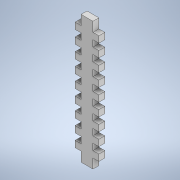
# Autodesk Inventor part: cover
Saved by Autodesk Inventor 2020 (Build 240168000, 168)
## iProperties
Created: 2019-12-19
Part Number: cover
Material: Générique
Document SubType Name: Modeling
Designer: damien
Density: 1 g/cm^3
Appearance: Par défaut
Author: damien
Autodesk Inventor part; units mm, degrees
ref_plane "YZ Plane" through (0, 0, 0) normal (1, 0, 0) x (0, 1, 0)
ref_plane "XZ Plane" through (0, 0, 0) normal (0, 1, 0) x (-1, 0, 0)
ref_plane "XY Plane" through (0, 0, 0) normal (0, 0, 1) x (1, 0, 0)
sketch "Esquisse1" plane through (0, 0, 0) normal (0, 0, 1) x (1, 0, 0)
  line L0 (37.1, -200) -> (-37.1, -200)
  line L1 (-37.1, -200) -> (-37.1, 200)
  line L2 (-37.1, 200) -> (37.1, 200)
  line L3 (37.1, 200) -> (37.1, -200)
  line L4 (37.1, -200) -> (-37.1, 200) construction
  line L5 (-37.1, -200) -> (37.1, 200) construction
  point P0 (0, 0)
  dimension "d0" = 400
  dimension "d1" = 74.2
  constraints: 12 end point, 2 midpoint, 2 parallel, 1 horizontal, 1 perpendicular
  measures "d0" distance of L0.end L1.end
  measures "d1" distance of L0.start L0.end
extrude "Extrusion1" add sketch "Esquisse1" along normal blind 18.55
sketch "Esquisse2" plane through (0, 0, 18.55) normal (0, 0, 1) x (1, 0, 0)
  line L0 (-37.1, 200) -> (-37.1, -200) projected
  line L1 (-37.1, 150) -> (-18.55, 150)
  line L2 (-18.55, 150) -> (-18.55, 130)
  line L3 (-18.55, 130) -> (-37.1, 130)
  line L4 (-37.1, 130) -> (-37.1, 150)
  line L5 (37.1, 200) -> (-37.1, 200) projected
  line L6 (-37.1, 90) -> (-37.1, 110)
  line L7 (-37.1, 110) -> (-18.55, 110)
  line L8 (-18.55, 110) -> (-18.55, 90)
  line L9 (-18.55, 90) -> (-37.1, 90)
  line L10 (-37.1, 50) -> (-37.1, 70)
  line L11 (-37.1, 70) -> (-18.55, 70)
  line L12 (-18.55, 70) -> (-18.55, 50)
  line L13 (-18.55, 50) -> (-37.1, 50)
  line L14 (-37.1, 10) -> (-37.1, 30)
  line L15 (-37.1, 30) -> (-18.55, 30)
  line L16 (-18.55, 30) -> (-18.55, 10)
  line L17 (-18.55, 10) -> (-37.1, 10)
  line L18 (-37.1, -30) -> (-37.1, -10)
  line L19 (-37.1, -10) -> (-18.55, -10)
  line L20 (-18.55, -10) -> (-18.55, -30)
  line L21 (-18.55, -30) -> (-37.1, -30)
  line L22 (-37.1, -70) -> (-37.1, -50)
  line L23 (-37.1, -50) -> (-18.55, -50)
  line L24 (-18.55, -50) -> (-18.55, -70)
  line L25 (-18.55, -70) -> (-37.1, -70)
  line L26 (-37.1, -110) -> (-37.1, -90)
  line L27 (-37.1, -90) -> (-18.55, -90)
  line L28 (-18.55, -90) -> (-18.55, -110)
  line L29 (-18.55, -110) -> (-37.1, -110)
  line L30 (-37.1, -150) -> (-37.1, -130)
  line L31 (-37.1, -130) -> (-18.55, -130)
  line L32 (-18.55, -130) -> (-18.55, -150)
  line L33 (-18.55, -150) -> (-37.1, -150)
  line L34 (-37.1, 200) -> (-18.55, 200)
  line L35 (-18.55, 200) -> (-18.55, 170)
  line L36 (-18.55, 170) -> (-37.1, 170)
  line L37 (-37.1, 170) -> (-37.1, 200)
  line L38 (-37.1, -200) -> (37.1, -200) projected
  line L39 (-37.1, -200) -> (-18.55, -200)
  line L40 (-18.55, -200) -> (-18.55, -170)
  line L41 (-18.55, -170) -> (-37.1, -170)
  line L42 (-37.1, -170) -> (-37.1, -200)
  point P0 (0, 0)
  point P1 (-37.1, -130)
  point P2 (-37.1, -150)
  point P3 (-37.1, -90)
  point P4 (-37.1, -110)
  point P5 (-37.1, -50)
  point P6 (-37.1, -10)
  point P7 (-37.1, -30)
  point P8 (-37.1, 70)
  point P9 (-37.1, 50)
  point P10 (-37.1, 110)
  dimension "d6" = 20
  dimension "d7" = 18.55
  dimension "d10" = 40
  dimension "d17" = 30
  dimension "d18" = 20
  dimension "d19" = 30
  constraints: 80 end point, 6 parallel, 3 horizontal, 3 perpendicular, 2 collinear, 1 point on line, 1 vertical, 56 other
  measures "d6" distance of L1.end L2.end
  measures "d7" distance of L1.start L1.end
  measures "d10" distance of L3.end L6.start
  measures "d17" distance of L36.end L0.start
  measures "d18" distance between parallel lines of L1 L36
  measures "d19" distance of L39.end L40.end
extrude "Extrusion2" cut sketch "Esquisse2" against normal blind 18.55
mirror "Symétrie1" about plane through (0, 0, 0) normal (1, 0, 0) of "Extrusion2"
